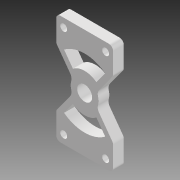
# Autodesk Inventor part: 2104_Tx_CoilBackPlate_V1
Saved by Autodesk Inventor 2021 (Build 250183000, 183)
## iProperties
Created: 2022-08-11
Part Number: 2104_Tx_CoilBackPlate_V1
Material: Generic
Document SubType Name: Modeling
Designer: Eli
Density: 1 g/cm^3
Appearance: Default
Author: Eli
Autodesk Inventor part; units mm, degrees
ref_plane "YZ Plane" through (0, 0, 0) normal (1, 0, 0) x (0, 1, 0)
ref_plane "XZ Plane" through (0, 0, 0) normal (0, 1, 0) x (-1, 0, 0)
ref_plane "XY Plane" through (0, 0, 0) normal (0, 0, 1) x (1, 0, 0)
sketch "Sketch1" plane through (0, 0, 0) normal (0, 0, 1) x (1, 0, 0)
  circle A0 centre (9.7751, -3.2289) radius 1.621 projected
  circle A1 centre (-9.7751, -3.2289) radius 1.621 projected
  line L0 (-11.2751, -7.2289) -> (11.2751, -7.2289) projected
  line L1 (13.2751, -5.2289) -> (13.2751, 4.1213) projected
  line L2 (12.8932, 5.2968) -> (12.7957, 5.4309) projected
  line L3 (-12.7957, 5.4309) -> (-12.8932, 5.2968) projected
  line L4 (-13.2751, 4.1213) -> (-13.2751, -5.2289) projected
  circle A2 centre (-9.7751, 39.9572) radius 1.621 projected
  circle A3 centre (9.7751, 39.9572) radius 1.621 projected
  line L5 (11.2751, 43.9572) -> (-11.2751, 43.9572) projected
  line L6 (-13.2751, 41.9572) -> (-13.2751, 32.607) projected
  line L7 (-12.8932, 31.4315) -> (-12.7957, 31.2974) projected
  line L8 (12.7957, 31.2974) -> (12.8932, 31.4315) projected
  line L9 (13.2751, 32.607) -> (13.2751, 41.9572) projected
  line L10 (13.2751, -7.2289) -> (-13.2751, -7.2289)
  line L11 (-13.2751, -7.2289) -> (-13.2751, 43.9572)
  line L12 (-13.2751, 43.9572) -> (13.2751, 43.9572)
  line L13 (13.2751, 43.9572) -> (13.2751, -7.2289)
  circle A4 centre (0, 18.3641) radius 3.5
  circle A5 centre (0, 18.3641) radius 6.5
  line L14 (13.2751, 31.9572) -> (5.6866, 21.5125)
  line L15 (13.2751, 4.7711) -> (5.6866, 15.2158)
  line L16 (-13.2751, 4.7711) -> (-5.6866, 15.2158)
  line L17 (-13.2751, 31.9572) -> (-5.6866, 21.5125)
  arc A6 (-11.4894, 7.2289) -> (11.4894, 7.2289) centre (0, 18.3641) ccw
  arc A7 (11.4894, 29.4994) -> (-11.4894, 29.4994) centre (0, 18.3641) ccw
  line L18 (5.6866, 15.2158) -> (11.4894, 7.2289)
  line L19 (-5.6866, 15.2158) -> (-11.4894, 7.2289)
  arc A8 (-5.6866, 15.2158) -> (5.6866, 15.2158) centre (0, 18.3641) ccw
  line L20 (5.4903, 11.2327) -> (9.6057, 5.5684)
  arc A9 (-5.4903, 11.2327) -> (5.4903, 11.2327) centre (0, 18.3641) ccw
  line L21 (-9.6057, 5.5684) -> (-5.4903, 11.2327)
  line L22 (0, 18.3641) -> (-13.2751, 18.3641) construction
  circle A10 centre (0, 18.3641) radius 6.5 construction
  arc A11 (5.6866, 21.5125) -> (-5.6866, 21.5125) centre (0, 18.3641) ccw
  line L23 (5.4903, 25.4955) -> (9.6057, 31.1599)
  arc A12 (5.4903, 25.4955) -> (-5.4903, 25.4955) centre (0, 18.3641) ccw
  line L24 (-9.6057, 31.1599) -> (-4.02, 23.4719)
  arc A13 (-13.2751, 32.607) -> (-12.8932, 31.4315) centre (-11.2751, 32.607) ccw projected
  arc A14 (-12.7957, 31.2974) -> (-12.6739, 31.1458) centre (-11.1777, 32.473) ccw projected
  arc A15 (12.6739, 31.1458) -> (-12.6739, 31.1458) centre (0, 18.3641) ccw projected
  arc A16 (12.6739, 31.1458) -> (12.7957, 31.2974) centre (11.1777, 32.473) ccw projected
  arc A17 (12.8932, 31.4315) -> (13.2751, 32.607) centre (11.2751, 32.607) ccw projected
  arc A18 (13.2751, 41.9572) -> (11.2751, 43.9572) centre (11.2751, 41.9572) ccw projected
  arc A19 (-11.2751, 43.9572) -> (-13.2751, 41.9572) centre (-11.2751, 41.9572) ccw projected
  arc A20 (13.2751, 4.1213) -> (12.8932, 5.2968) centre (11.2751, 4.1213) ccw projected
  arc A21 (12.7957, 5.4309) -> (12.6739, 5.5825) centre (11.1777, 4.2553) ccw projected
  arc A22 (-12.6739, 5.5825) -> (12.6739, 5.5825) centre (0, 18.3641) ccw projected
  arc A23 (-12.6739, 5.5825) -> (-12.7957, 5.4309) centre (-11.1777, 4.2553) ccw projected
  arc A24 (-12.8932, 5.2968) -> (-13.2751, 4.1213) centre (-11.2751, 4.1213) ccw projected
  arc A25 (-13.2751, -5.2289) -> (-11.2751, -7.2289) centre (-11.2751, -5.2289) ccw projected
  arc A26 (11.2751, -7.2289) -> (13.2751, -5.2289) centre (11.2751, -5.2289) ccw projected
  point P0 (0, 0)
  point P1 (8.136, 7.5912)
  point P2 (-8.136, 7.5912)
  point P3 (8.136, 29.1371)
  point P4 (-8.136, 29.1371)
  dimension "d0" = 7
  dimension "d1" = 13
  dimension "d4" = 2.5
  dimension "d5" = 2.5
  dimension "d6" = 2.5
  constraints: 30 end point, 23 point on circle, 9 centre point, 6 point on line, 5 collinear, 4 symmetric about line, 2 coincident, 2 horizontal, 2 parallel, 1 concentric, 1 midpoint, 1 perpendicular, 3 other
  measures "d0" diameter of A4
  measures "d1" diameter of A5
  measures "d4" distance between parallel lines of L18 L20
  measures "d5" radial gap between concentric circles of A8 A9
  measures "d6" distance between parallel lines of L19 L21
extrude "Extrusion1" add sketch "Sketch1" along normal blind 5 contours A25 L4 A24 L3 A23 A22 A21 L2 A20 L1 A26 L0 | L16 A6 L15 A21 A22 A23 | L6 A19 L5 A18 L9 A17 L8 A16 A15 A14 L7 A13 | L16 A5 L15 A6 L20 A9 L21 | A14 A15 A16 L14 A7 L17 | A5 | A7 L24 A5 L17 | L14 A5 L24 A12 L23 A7
fillet "Fillet1" radius 3.175 4 edges at (5.6866, 15.2158, 2.5) (5.6866, 21.5125, 2.5) (-5.6866, 15.2158, 2.5) (-5.6866, 21.5125, 2.5)
sketch "Sketch2" plane through (0, 0, 5) normal (0, 0, 1) x (1, 0, 0)
  circle A0 centre (9.7751, -3.2289) radius 1.621 projected
  circle A1 centre (-9.7751, -3.2289) radius 1.621 projected
  circle A2 centre (9.7751, 39.9572) radius 1.621 projected
  circle A3 centre (-9.7751, 39.9572) radius 1.621 projected
  circle A4 centre (9.7751, -3.2289) radius 1.621 projected
  circle A5 centre (-9.7751, -3.2289) radius 1.621 projected
  point P0 (0, 0)
  constraints: 4 coincident
hole "Hole1" at (9.7751, -3.2289, 5) at (-9.7751, -3.2289, 5) at (-9.7751, 39.9572, 5) at (9.7751, 39.9572, 5) direction (0, 0, -1) diameter 4.4958 end through all clearance for "Flat Head Machine Screw" size "M4" standard "Ansi Metric M Profile"
body "Solid1"
